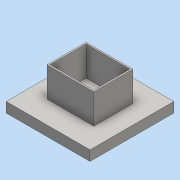
# Autodesk Inventor part: RJ45_bulkhead
Saved by Autodesk Inventor 2016 (Build 200138000, 138)
## iProperties
Created: 2016-09-22
Part Number: RJ45_bulkhead
Material: Generic
Document SubType Name: Modeling
Designer: Zara
Density: 1 g/cm^3
Appearance: Default
Author: Zara
Autodesk Inventor part; units mm, degrees
ref_plane "YZ Plane" through (0, 0, 0) normal (1, 0, 0) x (0, 1, 0)
ref_plane "XZ Plane" through (0, 0, 0) normal (0, 1, 0) x (-1, 0, 0)
ref_plane "XY Plane" through (0, 0, 0) normal (0, 0, 1) x (1, 0, 0)
sketch "Sketch1" plane through (0, 0, 0) normal (0, 0, 1) x (1, 0, 0)
  line L0 (-17.15, -17.15) -> (17.15, -17.15)
  line L1 (17.15, -17.15) -> (17.15, 17.15)
  line L2 (17.15, 17.15) -> (-17.15, 17.15)
  line L3 (-17.15, 17.15) -> (-17.15, -17.15)
  line L4 (-17.15, -17.15) -> (17.15, 17.15) construction
  line L5 (17.15, -17.15) -> (-17.15, 17.15) construction
  point P0 (0, 0)
  dimension "d0" = 34.3
  dimension "d1" = 34.3
  constraints: 12 end point, 2 midpoint, 2 parallel, 1 horizontal, 1 perpendicular
  measures "d0" distance of L1.end L2.end
  measures "d1" distance of L0.end L1.end
extrude "Extrusion1" add sketch "Sketch1" along normal blind 4.15
sketch "Sketch2" plane through (0, 0, 4.15) normal (0, 0, 1) x (1, 0, 0)
  line L0 (-9.025, -7.45) -> (9.025, -7.45)
  line L1 (9.025, -7.45) -> (9.025, 7.45)
  line L2 (9.025, 7.45) -> (-9.025, 7.45)
  line L3 (-9.025, 7.45) -> (-9.025, -7.45)
  line L4 (-9.025, -7.45) -> (9.025, 7.45) construction
  line L5 (9.025, -7.45) -> (-9.025, 7.45) construction
  line L6 (-9.5751, 8.0001) -> (9.5751, 8.0001)
  line L7 (9.5751, 8.0001) -> (9.5751, -8.0001)
  line L8 (9.5751, -8.0001) -> (-9.5751, -8.0001)
  line L9 (-9.5751, -8.0001) -> (-9.5751, 8.0001)
  point P0 (0, 0)
  dimension "d4" = 18.05
  dimension "d5" = 14.9
  constraints: 20 end point, 4 parallel, 2 midpoint, 2 perpendicular, 1 horizontal, 3 other
  measures "d4" distance of L1.end L2.end
  measures "d5" distance of L0.end L1.end
extrude "Extrusion2" add sketch "Sketch2" along normal blind 12.25
body "Solid1"
